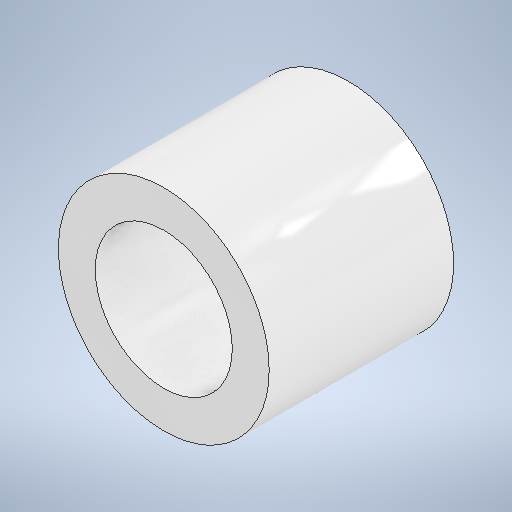
# Autodesk Inventor part: spacer 3.5mm
Saved by Autodesk Inventor 2025.2 (Build 292293000, 293)
## iProperties
Category: <PART CATAGORY>
Created: 2025-01-21
Part Number: spacer 3.5mm
Material: Generic
Document SubType Name: Modeling
Designer: lachl
Density: 1 g/cm^3
Appearance: Default
Title: <TITLE>
Author: lachl
Revision Number: 1
Autodesk Inventor part; units mm, degrees
ref_plane "YZ Plane" through (0, 0, 0) normal (1, 0, 0) x (0, 1, 0)
ref_plane "XZ Plane" through (0, 0, 0) normal (0, 1, 0) x (-1, 0, 0)
ref_plane "XY Plane" through (0, 0, 0) normal (0, 0, 1) x (1, 0, 0)
sketch "Sketch6" plane through (0, 0, 0) normal (0, 0, 1) x (1, 0, 0)
  circle A0 centre (-0.958, 0.7738) radius 1.3
  circle A1 centre (-0.958, 0.7738) radius 2
  point P0 (0, 0)
  dimension "d85" = 4
  dimension "d86" = 2.6
  constraints: 2 centre point, 1 concentric
  measures "d85" diameter of A1
  measures "d86" diameter of A0
extrude "Extrusion3" add sketch "Sketch6" along normal blind 3.5
body "Solid2"
